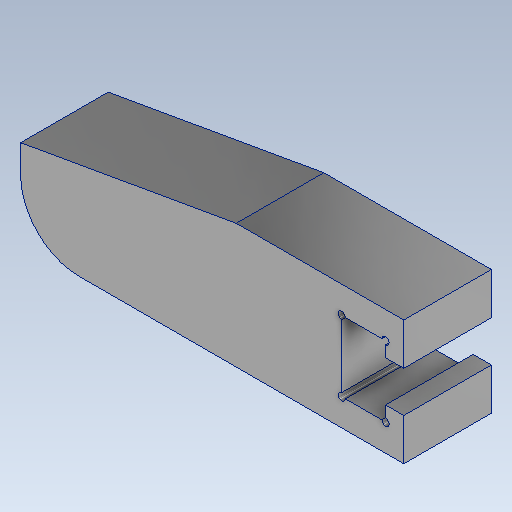
# Autodesk Inventor part: Finray_9_Kerbe_10deg_anschluss_erweitert_9_75 Nut
Saved by Autodesk Inventor 2025.2 (Build 292293000, 293)
## iProperties
Created: 2022-02-28
Part Number: Finray_9_Kerbe_10deg_anschluss_erweitert_9_75 Nut
Material: Generic
Document SubType Name: Modeling
Designer: richa
Density: 1 g/cm^3
Appearance: Aluminum - Flat
Author: richa
## iProperties of the stored document Maria_Greifer_Dreieck2_3D-Druck.ipt
Created: 2024-11-23
Part Number: Maria_Greifer_Dreieck2_3D-Druck
Material: Generisch
Document SubType Name: Modeling
Designer: maria
Density: 1 g/cm^3
Appearance: Vorgabe
Author: maria
Autodesk Inventor part; units mm, degrees
ref_plane "YZ Plane" through (0, 0, 0) normal (1, 0, 0) x (0, 1, 0)
ref_plane "XZ Plane" through (0, 0, 0) normal (0, 1, 0) x (-1, 0, 0)
ref_plane "XY Plane" through (0, 0, 0) normal (0, 0, 1) x (1, 0, 0)
sketch "Sketch5" plane through (0, 0, 0) normal (0, 0, 1) x (1, 0, 0)
  line L0 (52.5, -14.7318) -> (52.5, -9.0024)
  line L1 (52.5, -9.0024) -> (50, -9.0024)
  line L2 (50, -9.0024) -> (50, -11.0274)
  line L3 (44, -11.0274) -> (44, -1.3774)
  line L4 (50, -1.3774) -> (50, -3.4024)
  line L5 (50, -3.4024) -> (52.5, -3.4024)
  line L6 (52.5, -3.4024) -> (52.5, 2.327)
  line L7 (44, -1.3774) -> (50, -1.3774)
  line L8 (44, -11.0274) -> (50, -11.0274)
  line L9 (52.5, -14.7318) -> (44, -14.7318)
  line L10 (40.2429, -14.7318) -> (44, -14.7318)
  line L11 (0, -14.7318) -> (40.2429, -14.7318)
  line L12 (0, -14.7318) -> (0, -2.8824)
  line L13 (0, -2.8824) -> (29.5442, 2.327)
  line L14 (29.5442, 2.327) -> (52.5, 2.327)
  point P0 (0, 0)
  dimension "d41" = 6
  dimension "d48" = 44
  dimension "d50" = 2.5
  dimension "d87" = 5.6
  dimension "d88" = 9.65
  dimension "d115" = 10
  dimension "d116" = 30
  dimension "d117" = 0
  constraints: 30 end point, 6 perpendicular, 5 collinear, 3 horizontal, 2 parallel, 2 vertical
  measures "d41" distance between parallel lines of L2 L3
  measures "d48" distance from line of L3 point (0, 0)
  measures "d50" distance of L4.end L5.end
  measures "d87" distance from line of L0.end L5
  measures "d88" distance of L3.start L3.end
  measures "d115" angle of L13 L14
  measures "d116" distance of L12.end L13.end
  measures "d117" distance from line of L12 point (0, 0)
extrude "Extrusion2" add sketch "Sketch5" along normal blind 12
sketch "Sketch11" plane through (0, 0, 12) normal (0, 0, 1) x (1, 0, 0)
  line L0 (44, -1.3774) -> (50, -1.3774) projected
  circle A0 centre (44, -1.3774) radius 0.5
  line L1 (44, -11.0274) -> (44, -1.3774) projected
  circle A1 centre (44, -11.0274) radius 0.5
  line L2 (50, -11.0274) -> (44, -11.0274) projected
  circle A2 centre (50, -11.0274) radius 0.5
  line L3 (50, -1.3774) -> (50, -3.4024) projected
  circle A3 centre (50, -1.3774) radius 0.5
  point P0 (0, 0)
  dimension "d99" = 1
  dimension "d100" = 1
  dimension "d101" = 1
  dimension "d102" = 1
  constraints: 4 centre point, 1 coincident
  measures "d99" diameter of A0
  measures "d100" diameter of A1
  measures "d101" diameter of A2
  measures "d102" diameter of A3
extrude "Extrusion7" cut sketch "Sketch11" against normal through all
fillet "Rundung4" radius 8 1 edges at (0, -14.7318, 6)
equation "\"l1\" = 8"
body "Solid2"
